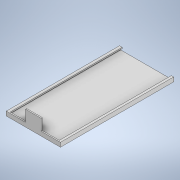
# Autodesk Inventor part: Deckel-Pumpe.v2
Saved by Autodesk Inventor 2020 (Build 240168000, 168)
## iProperties
Created: 2019-08-19
Part Number: Deckel-Pumpe.v2
Material: Generisch
Document SubType Name: Modeling
Designer: Admin
Density: 1 g/cm^3
Appearance: Vorgabe
Author: Admin
Autodesk Inventor part; units mm, degrees
ref_plane "YZ Plane" through (0, 0, 0) normal (1, 0, 0) x (0, 1, 0)
ref_plane "XZ Plane" through (0, 0, 0) normal (0, 1, 0) x (-1, 0, 0)
ref_plane "XY Plane" through (0, 0, 0) normal (0, 0, 1) x (1, 0, 0)
sketch "Skizze1" plane through (0, 0, 0) normal (0, 1, 0) x (-1, 0, 0)
  line L0 (0, 0) -> (63, 0)
  line L1 (63, 0) -> (63, 145)
  line L2 (63, 145) -> (0, 145)
  line L3 (0, 145) -> (0, 0)
  line L4 (63, 0) -> (67, 0)
  line L5 (63, 123.7495) -> (63, 0)
  line L6 (0, 0) -> (-4, 0)
  line L7 (0, 125) -> (0, 0)
  line L8 (63, 0) -> (66.5, 0)
  line L9 (66.5, 0) -> (66.5, 145)
  line L10 (66.5, 145) -> (63, 145)
  line L11 (63, 145) -> (63, 0)
  line L12 (66.5, 145) -> (65, 145)
  line L13 (65, 145) -> (65, 0)
  line L14 (65, 0) -> (66.5, 0)
  line L15 (66.5, 0) -> (66.5, 145)
  line L16 (0, 0) -> (-3.5, 0)
  line L17 (-3.5, 0) -> (-3.5, 145)
  line L18 (-3.5, 145) -> (0, 145)
  line L19 (0, 145) -> (0, 0)
  line L20 (-3.5, 0) -> (-2, 0)
  line L21 (-2, 0) -> (-2, 145)
  line L22 (-2, 145) -> (-3.5, 145)
  line L23 (-3.5, 145) -> (-3.5, 0)
  line L24 (66.5, 145) -> (-3.5, 145)
  line L25 (-3.5, 145) -> (-3.5, 146.5)
  line L26 (-3.5, 146.5) -> (66.5, 146.5)
  line L27 (66.5, 146.5) -> (66.5, 145)
  line L28 (41.5, 145) -> (21.5, 145)
  line L29 (21.5, 145) -> (21.5, 146.5)
  line L30 (21.5, 146.5) -> (41.5, 146.5)
  line L31 (41.5, 146.5) -> (41.5, 145)
  point P0 (65, 0)
  point P1 (0, 145)
  point P2 (-2, 0)
  point P3 (-3.5, 0)
  dimension "d0" = 63
  dimension "d1" = 145
  dimension "d5" = 1.5
  dimension "d6" = 3.5
  dimension "d7" = 3.5
  dimension "d8" = 1.5
  dimension "d9" = 1.5
  dimension "d29" = 0
  dimension "d31" = 0
  dimension "d32" = 0
  dimension "d33" = 20
  dimension "d34" = 25
  dimension "d35" = 25
  constraints: 64 end point, 14 parallel, 9 horizontal, 7 perpendicular, 4 point on line
  measures "d0" distance between parallel lines of L3 L1
  measures "d1" distance between parallel lines of L2 L0
  measures "d5" distance between parallel lines of L13 L9
  measures "d6" distance between parallel lines of L5 L9
  measures "d7" distance between parallel lines of L7 L17
  measures "d8" distance between parallel lines of L17 L21
  measures "d9" distance between parallel lines of L26 L2
  measures "d29" distance from line of L23 L24.end
  measures "d31" distance between parallel lines of L2 L24
  measures "d32" distance between parallel lines of L24 L18
  measures "d33" distance between parallel lines of L29 L31
  measures "d34" distance from line of L25 L28.end
  measures "d35" distance between parallel lines of L31 L27
extrude "Extrusion1" add sketch "Skizze1" along normal blind 1.5 contours L3 L2 L1 L0 | L6 L21 L18 L3 | L1 L10 L13 L4
extrude "Extrusion2" add sketch "Skizze1" along normal blind 4 contours L6 L17 L18 L21 | L13 L10 L9 L4
sketch "Skizze2" plane through (0, 4, 0) normal (0, 1, 0) x (1, 0, 0)
  line L0 (-66.5, -145) -> (3.5, -145) projected
  line L1 (2, 0) -> (-65, 0) projected
  line L2 (3.5, -145) -> (0.5, -145)
  line L3 (0.5, -145) -> (0.5, 0)
  line L4 (0.5, 0) -> (3.5, 0)
  line L5 (3.5, 0) -> (3.5, -145)
  point P0 (0, 0)
  point P1 (-63, -125)
  point P2 (2, 0)
  point P3 (0.5, -144.0977)
  dimension "d14" = 3
  constraints: 8 end point, 2 parallel, 1 horizontal, 1 perpendicular, 1 point on line, 1 other
  measures "d14" distance between parallel lines of L5 L3
extrude "Extrusion3" add sketch "Skizze2" along normal blind 1.5
sketch "Skizze3" plane through (0, 4, 0) normal (0, 1, 0) x (1, 0, 0)
  line L0 (-66.5, 0) -> (-66.5, -145) projected
  line L1 (-66.5, 0) -> (-63, 0)
  line L2 (-63, 0) -> (-63, -125.035)
  line L3 (-66.5, -125.035) -> (-66.5, 0)
  line L4 (-63, -125.035) -> (-63, -145)
  line L5 (-63, -145) -> (-66.5, -145)
  point P0 (0, 0)
  point P1 (-66.5, -125.035)
  dimension "d17" = 3.5
  constraints: 10 end point, 2 perpendicular, 1 horizontal, 1 parallel, 1 vertical
  measures "d17" distance between parallel lines of L0 L2
extrude "Extrusion4" add sketch "Skizze3" along normal blind 1.5
extrude "Extrusion5" add sketch "Skizze1" along normal blind 5.5 contours L18 L25 L26 L29 L2 | L2 L31 L26 L27 L10 | L29 L26 L31 L2
sketch "Skizze4" plane through (3.5, 0, 0) normal (0, 0, -1) x (-1, 0, 0)
  line L0 (1.5, 1.5) -> (68.5, 1.5) projected
  line L1 (0, 0) -> (70, 0) projected
  line L2 (1.5, 4) -> (3, 4) projected
  line L3 (0, 5.5) -> (3, 5.5) projected
  line L4 (0, 0) -> (0, 5.5) projected
  line L5 (3, 4) -> (3, 5.5) projected
  line L6 (1.5, 1.5) -> (1.5, 4) projected
  line L7 (68.5, 1.5) -> (68.5, 4) projected
  line L8 (66.5, 4) -> (66.5, 5.5) projected
  line L9 (70, 0) -> (70, 5.5) projected
  point P0 (3.5, 0)
  dimension "d22" = 1.5
  dimension "d23" = 2.5
  dimension "d24" = 1.5
  dimension "d25" = 3
  dimension "d26" = 1.5
  dimension "d27" = 67
  dimension "d28" = 63.5
  dimension "d30" = 70
  measures "d22" distance between parallel lines of L0 L1
  measures "d23" distance between parallel lines of L2 L0
  measures "d24" distance between parallel lines of L3 L2
  measures "d25" distance between parallel lines of L4 L5
  measures "d26" distance between parallel lines of L4 L6
  measures "d27" distance between parallel lines of L6 L7
  measures "d28" distance from line of L3.end L8
  measures "d30" distance between parallel lines of L4 L9
extrude "Extrusion6" add sketch "Skizze1" along normal blind 20 contours L29 L26 L31 L2
